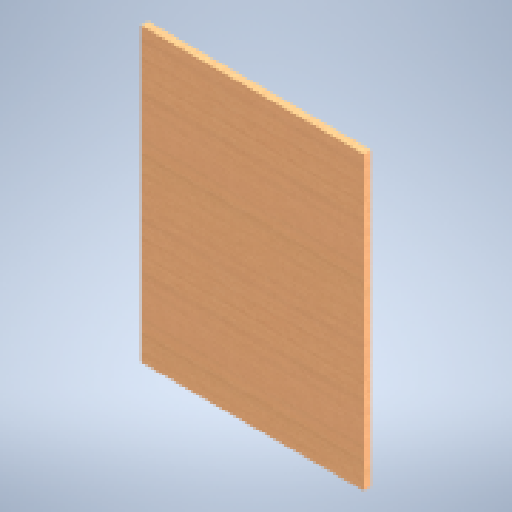
# Autodesk Inventor part: Rückseite_Gehäuse
Saved by Autodesk Inventor 2024 (Build 280153000, 153)
## iProperties
Created: 2024-03-12
Part Number: Rückseite_Gehäuse
Material: Holz (Kirsche)
Document SubType Name: Modeling
Designer: haniv
Density: 0.63 g/cm^3
Appearance: Kirsche - natur - schwacher Glanz
Author: haniv
Autodesk Inventor part; units mm, degrees
ref_plane "YZ Plane" through (0, 0, 0) normal (1, 0, 0) x (0, 1, 0)
ref_plane "XZ Plane" through (0, 0, 0) normal (0, 1, 0) x (-1, 0, 0)
ref_plane "XY Plane" through (0, 0, 0) normal (0, 0, 1) x (1, 0, 0)
sketch "Skizze1" plane through (0, 0, 0) normal (0, 1, 0) x (-1, 0, 0)
  line L0 (182, 238) -> (-182, 238)
  line L1 (-182, 238) -> (-182, -238)
  line L2 (-182, -238) -> (182, -238)
  line L3 (182, -238) -> (182, 238)
  point P0 (0, 0)
  point P1 (0, 238)
  point P2 (182, 0)
  dimension "d0" = 364
  dimension "d1" = 476
  constraints: 8 end point, 2 midpoint, 2 parallel, 1 horizontal, 1 horizontal alignment, 1 perpendicular, 1 vertical alignment
  measures "d0" distance of L2.end L1.end
  measures "d1" distance of L2.end L0.start
extrude "Extrusion1" add sketch "Skizze1" along normal blind 12
